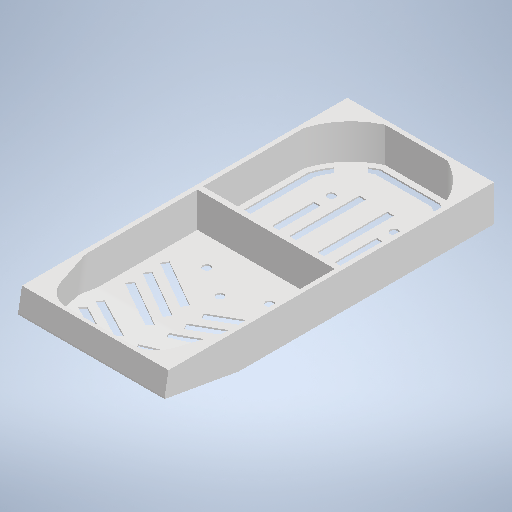
# Autodesk Inventor part: sole_paint_support
Saved by Autodesk Inventor 2026.1 (Build 301233020, 233B)
## iProperties
Created: 2026-02-24
Part Number: sole_paint_support
Material: 一般
Document SubType Name: Modeling
Designer: hibik
Density: 1 g/cm^3
Appearance: 既定
Author: hibik
Autodesk Inventor part; units mm, degrees
ref_plane "YZ Plane" through (0, 0, 0) normal (1, 0, 0) x (0, 1, 0)
ref_plane "XZ Plane" through (0, 0, 0) normal (0, 1, 0) x (-1, 0, 0)
ref_plane "XY Plane" through (0, 0, 0) normal (0, 0, 1) x (1, 0, 0)
sketch "スケッチ1" plane through (0, 0, 0) normal (0, 1, 0) x (-1, 0, 0)
  line L0 (-15.856406, 24.133975) -> (-5.024845, 30.387579)
  line L1 (5.024845, 30.387579) -> (-5.024845, 30.387579)
  line L2 (5.024845, 30.387579) -> (15.856406, 24.133975)
  line L3 (15.856406, 24.133975) -> (16.856406, 25.866025)
  line L4 (16.856406, 25.866025) -> (9.024845, 30.387579)
  line L5 (19, 30.387579) -> (9.024845, 30.387579)
  line L6 (19, 30.387579) -> (19, 3)
  line L7 (19, 3) -> (-19, 3)
  line L8 (-19, 3) -> (-19, 30.387579)
  line L9 (-9.024845, 30.387579) -> (-19, 30.387579)
  line L10 (-9.024845, 30.387579) -> (-16.856406, 25.866025)
  line L11 (-16.856406, 25.866025) -> (-15.856406, 24.133975)
  line L12 (2, 22.133975) -> (15.856406, 14.133975)
  line L13 (15.856406, 14.133975) -> (16.856406, 15.866025)
  line L14 (16.856406, 15.866025) -> (3, 23.866025)
  line L15 (3, 23.866025) -> (2, 22.133975)
  line L16 (2, 27.133975) -> (15.856406, 19.133975)
  line L17 (15.856406, 19.133975) -> (16.856406, 20.866025)
  line L18 (16.856406, 20.866025) -> (3, 28.866025)
  line L19 (3, 28.866025) -> (2, 27.133975)
  line L20 (-16.856406, 15.866025) -> (-15.856406, 14.133975)
  line L21 (-15.856406, 14.133975) -> (-2, 22.133975)
  line L22 (-2, 22.133975) -> (-3, 23.866025)
  line L23 (-3, 23.866025) -> (-16.856406, 15.866025)
  line L24 (-16.856406, 20.866025) -> (-15.856406, 19.133975)
  line L25 (-15.856406, 19.133975) -> (-2, 27.133975)
  line L26 (-2, 27.133975) -> (-3, 28.866025)
  line L27 (-3, 28.866025) -> (-16.856406, 20.866025)
  circle A0 centre (0, 15.5) radius 2.5
  circle A1 centre (-9, 10.307692) radius 2.5
  circle A2 centre (9, 10.307692) radius 2.5
  line L28 (19, -28.244998) -> (19, 0)
  arc A3 (8.717798, -40) -> (19, -28.244998) centre (0, -22) ccw
  line L29 (8.717798, -40) -> (-8.717798, -40)
  arc A4 (-19, -28.244998) -> (-8.717798, -40) centre (0, -22) ccw
  line L30 (-19, -28.244998) -> (-19, 0)
  line L31 (-19, 0) -> (19, 0)
  circle A5 centre (9, -25.384615) radius 2.5
  circle A6 centre (-9, -25.384615) radius 2.5
  circle A7 centre (-9, -4.615385) radius 2.5
  circle A8 centre (9, -4.615385) radius 2.5
  line L32 (-10, -21.384615) -> (-8, -21.384615)
  line L33 (-8, -21.384615) -> (-8, -8.615385)
  line L34 (-8, -8.615385) -> (-10, -8.615385)
  line L35 (-10, -8.615385) -> (-10, -21.384615)
  line L36 (18.05, -27.932748) -> (18.05, -1)
  line L37 (18.05, -1) -> (16.05, -1)
  line L38 (16.05, -1) -> (16.05, -27.603347)
  arc A9 (14.238164, -31.288417) -> (16.05, -27.603347) centre (0, -22) ccw
  line L39 (8, -37) -> (-8, -37)
  arc A10 (-16.05, -27.603347) -> (-14.238164, -31.288417) centre (0, -22) ccw
  line L40 (-16.05, -27.603347) -> (-16.05, -1)
  line L41 (-16.05, -1) -> (-18.05, -1)
  line L42 (-18.05, -1) -> (-18.05, -27.932748)
  arc A11 (15.679986, -32.730239) -> (18.05, -27.932748) centre (0, -22) ccw
  line L43 (-8.485281, -39) -> (8.485281, -39)
  arc A12 (-18.05, -27.932748) -> (-15.679986, -32.730239) centre (0, -22) ccw
  line L44 (-3, -1) -> (-5, -1)
  line L45 (-5, -1) -> (-5, -29.421937)
  line L46 (-5, -29.421937) -> (-3, -29.421937)
  line L47 (-3, -29.421937) -> (-3, -1)
  line L48 (8, -21.384615) -> (10, -21.384615)
  line L49 (10, -21.384615) -> (10, -8.615385)
  line L50 (10, -8.615385) -> (8, -8.615385)
  line L51 (8, -8.615385) -> (8, -21.384615)
  line L52 (5, -1) -> (3, -1)
  line L53 (3, -1) -> (3, -29.421937)
  line L54 (3, -29.421937) -> (5, -29.421937)
  line L55 (5, -29.421937) -> (5, -1)
  line L56 (21, 52.387579) -> (-21, 52.387579)
  line L57 (-21, 52.387579) -> (-21, -42)
  line L58 (-21, -42) -> (21, -42)
  line L59 (21, -42) -> (21, 52.387579)
  line L60 (9.024845, 30.387579) -> (-9.024845, 30.387579)
  line L61 (15.679986, -32.730239) -> (14.238164, -31.288417)
  line L62 (-15.679986, -32.730239) -> (-14.238164, -31.288417)
  line L63 (9.288417, -36.238164) -> (10.730239, -37.679986)
  arc A13 (8, -37) -> (9.288417, -36.238164) centre (0, -22) ccw
  arc A14 (-9.288417, -36.238164) -> (-8, -37) centre (0, -22) ccw
  line L64 (-9.288417, -36.238164) -> (-10.730239, -37.679986)
  arc A15 (-10.730239, -37.679986) -> (-8.485281, -39) centre (0, -22) ccw
  arc A16 (8.485281, -39) -> (10.730239, -37.679986) centre (0, -22) ccw
  point P0 (0, 0)
  point P1 (0, 52.387579)
  dimension "d0" = 2
  dimension "d1" = 2
  dimension "d2" = 22
  constraints: 10 end point, 2 horizontal, 2 parallel, 1 midpoint, 1 perpendicular, 1 vertical alignment
  measures "d0" distance between parallel lines of L58 L29
  measures "d1" distance between parallel lines of L57 L8
  measures "d2" distance between parallel lines of L56 L9
extrude "押し出し1" add sketch "スケッチ1" against normal blind 0.4 contours L0 L1 L2 L3 L4 L5 L6 L7 L8 L9 L10 L11 | A0 | A1 | A2 | A3 L29 A4 L30 L31 L28 | A5 | A6 | A7 | A8 | L59 L58 L57 L56
sketch "スケッチ2" plane through (0, 0, 0) normal (1, 0, 0) x (0, 1, 0)
  line L0 (2.641813, 45.982466) -> (1.055373, 36.985318)
  line L1 (0.670986, 34.805353) -> (1.055373, 36.985318)
  line L2 (0.670986, 34.805353) -> (0.106346, 31.603117)
  arc A0 (0.106346, 31.603117) -> (0, 30.387579) centre (7, 30.387579) ccw
  line L3 (2.641813, 45.982466) -> (3.472964, 50.696155)
  line L4 (0, 52.387579) -> (0, -42)
  line L5 (0, 52.387579) -> (3.771207, 52.387579)
  line L6 (3.771207, 52.387579) -> (3.472964, 50.696155)
  point P0 (0, 0)
  constraints: 4 end point, 1 collinear, 1 horizontal
extrude "押し出し2" add sketch "スケッチ2" along normal mid plane 42
sketch "スケッチ3" plane through (21, -0.4, 52.387579) normal (1, 0, 0) x (0, 0, -1)
  line L0 (20.784463, 0.506346) -> (0, 4.171207)
  line L1 (21.352584, 0) -> (0, 3.765037)
  line L2 (94.387579, 0) -> (0, 0)
  line L3 (0, 4.171207) -> (0, 0)
  point P0 (52.387579, 0.4)
  dimension "d7" = 0.4
  constraints: 2 end point, 2 point on line, 1 parallel
  measures "d7" distance between parallel lines of L1 L0
extrude "押し出し3" cut sketch "スケッチ3" against normal through all
sketch "スケッチ4" plane through (-21, -0.4, 31.034995) normal (0, -0.9848078, 0.1736482) x (1, 0, 0)
  line L0 (18, 16.88502) -> (19, 15.15297)
  line L1 (19, 15.15297) -> (6, 7.647416)
  line L2 (6, 7.647416) -> (5, 9.379467)
  line L3 (5, 9.379467) -> (18, 16.88502)
  line L4 (36, 7.647416) -> (23, 15.15297)
  line L5 (23, 15.15297) -> (24, 16.88502)
  line L6 (24, 16.88502) -> (37, 9.379467)
  line L7 (37, 9.379467) -> (36, 7.647416)
  line L8 (37, 4.379467) -> (36, 2.647416)
  line L9 (36, 2.647416) -> (23, 10.15297)
  line L10 (23, 10.15297) -> (24, 11.88502)
  line L11 (24, 11.88502) -> (37, 4.379467)
  line L12 (19, 10.15297) -> (6, 2.647416)
  line L13 (6, 2.647416) -> (5, 4.379467)
  line L14 (5, 4.379467) -> (18, 11.88502)
  line L15 (18, 11.88502) -> (19, 10.15297)
  line L16 (23.919473, 0.647416) -> (23, 1.186463)
  line L17 (23, 1.186463) -> (24, 2.945234)
  line L18 (24, 2.945234) -> (27.919473, 0.647416)
  line L19 (40, 0.647416) -> (27.919473, 0.647416)
  line L20 (40, 3.899052) -> (40, 0.647416)
  arc A0 (40, 3.899052) -> (39.640783, 6.112646) centre (33, 3.899052) ccw
  line L21 (36.595469, 15.24859) -> (39.640783, 6.112646)
  arc A1 (36.595469, 15.24859) -> (29.954685, 20.034995) centre (29.954685, 13.034995) ccw
  line L22 (29.954685, 20.034995) -> (12.045315, 20.034995)
  arc A2 (12.045315, 20.034995) -> (5.404531, 15.24859) centre (12.045315, 13.034995) ccw
  line L23 (2.359217, 6.112646) -> (5.404531, 15.24859)
  arc A3 (2.359217, 6.112646) -> (2, 3.899052) centre (9, 3.899052) ccw
  line L24 (2, 0.647416) -> (2, 3.899052)
  line L25 (14.080527, 0.647416) -> (2, 0.647416)
  line L26 (14.080527, 0.647416) -> (18, 2.945234)
  line L27 (18, 2.945234) -> (19, 1.186463)
  line L28 (19, 1.186463) -> (18.080527, 0.647416)
  line L29 (23.919473, 0.647416) -> (18.080527, 0.647416)
  line L30 (11.975155, -0.63758) -> (15.975155, -0.63758)
  line L31 (26.024845, -0.63758) -> (30.024845, -0.63758)
  line L32 (26.024845, -0.63758) -> (23.919473, 0.647416)
  line L33 (30.024845, -0.63758) -> (27.919473, 0.647416)
  line L34 (18.080527, 0.647416) -> (15.975155, -0.63758)
  line L35 (4.143594, -5.090442) -> (11.975155, -0.63758)
  line L36 (11.975155, -0.63758) -> (14.080527, 0.647416)
  point P0 (21, -30.494045)
  constraints: 8 end point
extrude "押し出し4" cut sketch "スケッチ4" against normal through all contours L0 L1 L2 L3 | L4 L5 L6 L7 | L8 L9 L10 L11 | L12 L13 L14 L15 | L16 L17 L18 L33 L31 L32 | L34 L30 L36 L26 L27 L28
sketch "スケッチ5" plane through (0, 0, 0) normal (0, 1, 0) x (1, 0, 0)
  line L0 (-19, 28.244998) -> (-19, 0)
  line L1 (-19, 0) -> (19, 0)
  line L2 (19, 0) -> (19, 28.244998)
  arc A0 (19, 28.244998) -> (8.717798, 40) centre (0, 22) ccw
  line L3 (8.717798, 40) -> (-8.717798, 40)
  arc A1 (-8.717798, 40) -> (-19, 28.244998) centre (0, 22) ccw
  circle A2 centre (9, 25.384615) radius 0.8
  circle A3 centre (-9, 25.384615) radius 0.8
  circle A4 centre (9, 4.615385) radius 0.8
  circle A5 centre (-9, 4.615385) radius 0.8
  line L4 (19, -30.037625) -> (-19, -30.037625)
  line L5 (19, -30.037625) -> (19, -3)
  line L6 (19, -3) -> (-19, -3)
  line L7 (-19, -3) -> (-19, -30.037625)
  circle A6 centre (-9, -10.307692) radius 0.8
  circle A7 centre (9, -10.307692) radius 0.8
  circle A8 centre (0, -15.5) radius 0.8
  arc A9 (19.7, 28.356099) -> (8.876936, 40.7) centre (0, 22) ccw
  line L8 (19.7, 28.356099) -> (19.7, -0.7)
  line L9 (19.7, -0.7) -> (-19.7, -0.7)
  line L10 (-19.7, -0.7) -> (-19.7, 28.356099)
  arc A10 (-8.876936, 40.7) -> (-19.7, 28.356099) centre (0, 22) ccw
  line L11 (-8.876936, 40.7) -> (8.876936, 40.7)
  line L12 (19.7, -2.3) -> (19.7, -30.737625)
  line L13 (19.7, -30.737625) -> (-19.7, -30.737625)
  line L14 (-19.7, -30.737625) -> (-19.7, -2.3)
  line L15 (-19.7, -2.3) -> (19.7, -2.3)
  line L16 (-5, 1) -> (-5, 29.421937)
  line L17 (-5, 29.421937) -> (-3, 29.421937)
  line L18 (-3, 29.421937) -> (-3, 1)
  line L19 (-3, 1) -> (-5, 1)
  line L20 (-8, 21.384615) -> (-8, 8.615385)
  line L21 (-8, 8.615385) -> (-10, 8.615385)
  line L22 (-10, 8.615385) -> (-10, 21.384615)
  line L23 (-10, 21.384615) -> (-8, 21.384615)
  line L24 (3, 1) -> (3, 29.421937)
  line L25 (3, 29.421937) -> (5, 29.421937)
  line L26 (5, 29.421937) -> (5, 1)
  line L27 (5, 1) -> (3, 1)
  line L28 (10, 21.384615) -> (10, 8.615385)
  line L29 (10, 8.615385) -> (8, 8.615385)
  line L30 (8, 8.615385) -> (8, 21.384615)
  line L31 (8, 21.384615) -> (10, 21.384615)
  line L32 (16.856406, -20.866025) -> (3, -28.866025)
  line L33 (3, -28.866025) -> (2, -27.133975)
  line L34 (2, -27.133975) -> (15.856406, -19.133975)
  line L35 (15.856406, -19.133975) -> (16.856406, -20.866025)
  line L36 (16.856406, -15.866025) -> (3, -23.866025)
  line L37 (3, -23.866025) -> (2, -22.133975)
  line L38 (2, -22.133975) -> (15.856406, -14.133975)
  line L39 (15.856406, -14.133975) -> (16.856406, -15.866025)
  line L40 (-2, -27.133975) -> (-3, -28.866025)
  line L41 (-3, -28.866025) -> (-16.856406, -20.866025)
  line L42 (-16.856406, -20.866025) -> (-15.856406, -19.133975)
  line L43 (-15.856406, -19.133975) -> (-2, -27.133975)
  line L44 (-2, -22.133975) -> (-3, -23.866025)
  line L45 (-3, -23.866025) -> (-16.856406, -15.866025)
  line L46 (-16.856406, -15.866025) -> (-15.856406, -14.133975)
  line L47 (-15.856406, -14.133975) -> (-2, -22.133975)
  line L48 (-5.147008, -30.317049) -> (-5.024845, -30.317049)
  line L49 (-5.024845, -30.317049) -> (-4.911041, -30.387579)
  line L50 (4.911041, -30.387579) -> (-4.911041, -30.387579)
  line L51 (4.911041, -30.387579) -> (5.024845, -30.317049)
  line L52 (5.024845, -30.317049) -> (5.147008, -30.317049)
  line L53 (5.147008, -30.317049) -> (15.856406, -24.133975)
  line L54 (15.856406, -24.133975) -> (16.856406, -25.866025)
  line L55 (16.856406, -25.866025) -> (9.024845, -30.387579)
  line L56 (21, -30.387579) -> (9.024845, -30.387579)
  line L57 (21, -30.387579) -> (21, 42)
  line L58 (21, 42) -> (-21, 42)
  line L59 (-21, 42) -> (-21, -30.387579)
  line L60 (-9.024845, -30.387579) -> (-21, -30.387579)
  line L61 (-9.024845, -30.387579) -> (-16.856406, -25.866025)
  line L62 (-16.856406, -25.866025) -> (-15.856406, -24.133975)
  line L63 (-15.856406, -24.133975) -> (-5.147008, -30.317049)
  point P0 (0, 0)
  point P1 (19.7, -30.387579)
  point P2 (-19.7, -30.387579)
  dimension "d12" = 0.7
  dimension "d13" = 0.7
  constraints: 16 end point, 4 point on circle, 2 centre point, 8 other
  measures "d12" radial gap between concentric circles of A0 A9
  measures "d13" distance between parallel lines of L5 L12
extrude "押し出し5" add sketch "スケッチ5" along normal blind 10 contours L12 L15 L14 L60 L59 L58 L57 L56
sketch "スケッチ6" plane through (-21, 3.771207, 52.387579) normal (0, 0.9848078, -0.1736482) x (1, 0, 0)
  line L0 (2, 20.755142) -> (40, 20.755142)
  line L1 (2, 17.853461) -> (2, 20.755142)
  arc A0 (2, 17.853461) -> (2.359217, 15.639867) centre (9, 17.853461) ccw
  line L2 (5.404531, 6.503923) -> (2.359217, 15.639867)
  arc A1 (5.404531, 6.503923) -> (12.045315, 1.717517) centre (12.045315, 8.717517) ccw
  line L3 (29.954685, 1.717517) -> (12.045315, 1.717517)
  arc A2 (29.954685, 1.717517) -> (36.595469, 6.503923) centre (29.954685, 8.717517) ccw
  line L4 (39.640783, 15.639867) -> (36.595469, 6.503923)
  arc A3 (39.640783, 15.639867) -> (40, 17.853461) centre (33, 17.853461) ccw
  line L5 (40, 20.755142) -> (40, 17.853461)
  arc A4 (29.954685, 1.017517) -> (37.259547, 6.282563) centre (29.954685, 8.717517) ccw
  line L6 (29.954685, 1.017517) -> (12.045315, 1.017517)
  arc A5 (4.740453, 6.282563) -> (12.045315, 1.017517) centre (12.045315, 8.717517) ccw
  line L7 (4.740453, 6.282563) -> (1.695139, 15.418507)
  arc A6 (1.3, 17.853461) -> (1.695139, 15.418507) centre (9, 17.853461) ccw
  line L8 (1.3, 17.853461) -> (1.3, 21.455142)
  line L9 (1.3, 21.455142) -> (40.7, 21.455142)
  line L10 (40.7, 21.455142) -> (40.7, 17.853461)
  arc A7 (40.304861, 15.418507) -> (40.7, 17.853461) centre (33, 17.853461) ccw
  line L11 (40.304861, 15.418507) -> (37.259547, 6.282563)
  line L12 (18, 18.807279) -> (14.080527, 21.105097)
  line L13 (14.080527, 21.105097) -> (0, 21.105097)
  line L14 (0, 0) -> (0, 21.105097)
  line L15 (0, 0) -> (42, 0)
  line L16 (42, 21.105097) -> (42, 0)
  line L17 (42, 21.105097) -> (27.919473, 21.105097)
  line L18 (27.919473, 21.105097) -> (24, 18.807279)
  line L19 (24, 18.807279) -> (23, 20.566049)
  line L20 (23, 20.566049) -> (23.919473, 21.105097)
  line L21 (23.919473, 21.105097) -> (18.080527, 21.105097)
  line L22 (18.080527, 21.105097) -> (19, 20.566049)
  line L23 (19, 20.566049) -> (18, 18.807279)
  line L24 (5, 17.373046) -> (6, 19.105097)
  line L25 (6, 19.105097) -> (19, 11.599543)
  line L26 (19, 11.599543) -> (18, 9.867492)
  line L27 (18, 9.867492) -> (5, 17.373046)
  line L28 (24, 4.867492) -> (23, 6.599543)
  line L29 (23, 6.599543) -> (36, 14.105097)
  line L30 (36, 14.105097) -> (37, 12.373046)
  line L31 (37, 12.373046) -> (24, 4.867492)
  line L32 (6, 14.105097) -> (19, 6.599543)
  line L33 (19, 6.599543) -> (18, 4.867492)
  line L34 (18, 4.867492) -> (5, 12.373046)
  line L35 (5, 12.373046) -> (6, 14.105097)
  line L36 (23, 11.599543) -> (36, 19.105097)
  line L37 (36, 19.105097) -> (37, 17.373046)
  line L38 (37, 17.373046) -> (24, 9.867492)
  line L39 (24, 9.867492) -> (23, 11.599543)
  point P0 (21, 52.246558)
  point P1 (1.3, 21.105097)
  point P2 (40.7, 21.105097)
  dimension "d16" = 0.7
  constraints: 12 end point, 8 point on circle, 4 centre point, 9 other
  measures "d16" distance between parallel lines of L4 L11
extrude "押し出し6" add sketch "スケッチ6" along normal blind 10 contours L8 A6 L7 A5 L6 A4 L11 A7 L10 L17 L16 L15 L14 L13
sketch "スケッチ7" plane through (-21, -0.4, -42) normal (-1, 0, 0) x (0, 0, 1)
  line L0 (73.603117, 0.506346) -> (72.387579, 7.4)
  arc A0 (72.387579, 0.4) -> (73.603117, 0.506346) centre (72.387579, 7.4) ccw
  line L1 (72.387579, 0.4) -> (72.387579, 7.4)
  line L2 (73.603117, 0.506346) -> (72.387579, 7.4)
  line L3 (94.387579, 4.171207) -> (92.651098, 14.019285)
  line L4 (72.125113, 10.4) -> (92.651098, 14.019285)
  line L5 (0, 10.4) -> (72.125113, 10.4)
  line L6 (0, 0) -> (0, 10.4)
  line L7 (73.034995, 0) -> (0, 0)
  line L8 (73.034995, 0) -> (94.387579, 3.765037)
  line L9 (94.387579, 3.765037) -> (94.387579, 4.171207)
  point P0 (42, 0.4)
extrude "押し出し7" add sketch "スケッチ7" against normal up to surface (1.3 mm away) contours A0 L1 L0
sketch "スケッチ8" plane through (21, -0.4, 31.034995) normal (1, 0, 0) x (0, 0, -1)
  line L0 (-21.352584, 4.171207) -> (-21.352584, 3.765037)
  line L1 (-21.352584, 3.765037) -> (0, 0)
  line L2 (73.034995, 0) -> (0, 0)
  line L3 (73.034995, 0) -> (73.034995, 10.4)
  line L4 (0.909882, 10.4) -> (73.034995, 10.4)
  line L5 (-19.616102, 14.019285) -> (0.909882, 10.4)
  line L6 (-21.352584, 4.171207) -> (-19.616102, 14.019285)
  line L7 (-0.568121, 0.506346) -> (0.647416, 7.4)
  line L8 (0.647416, 0.4) -> (0.647416, 7.4)
  arc A0 (-0.568121, 0.506346) -> (0.647416, 0.4) centre (0.647416, 7.4) ccw
  point P0 (31.034995, 0.4)
extrude "押し出し8" add sketch "スケッチ8" against normal up to surface (1.3 mm away) contours L7 L8 A0
sketch "スケッチ9" plane through (0, 10, 0) normal (0, 1, 0) x (1, 0, 0)
  line L0 (50.426024, -14.988478) -> (-44.417108, -14.988478)
  line L1 (-44.417108, -14.988478) -> (-44.417108, -64.562339)
  line L2 (-44.417108, -64.562339) -> (50.426024, -64.562339)
  line L3 (50.426024, -64.562339) -> (50.426024, -14.988478)
  point P0 (0, 0)
  constraints: 8 end point, 2 parallel, 1 horizontal, 1 perpendicular
extrude "押し出し9" cut sketch "スケッチ9" along normal through all
sketch "スケッチ10" plane through (0, -0.4, 0) normal (0, -1, 0) x (1, 0, 0)
  circle A0 centre (9, -4.615385) radius 2.5
  circle A1 centre (-9, -4.615385) radius 2.5
  circle A2 centre (-9, -25.384615) radius 2.5
  circle A3 centre (9, -25.384615) radius 2.5
  circle A4 centre (9, 10.307692) radius 2.5
  circle A5 centre (-9, 10.307692) radius 2.5
  circle A6 centre (0, 15.5) radius 2.5
  circle A7 centre (9, -25.384615) radius 1.15
  circle A8 centre (-9, -25.384615) radius 1.15
  circle A9 centre (9, -4.615385) radius 1.15
  circle A10 centre (-9, -4.615385) radius 1.15
  circle A11 centre (-9, 10.307692) radius 1.15
  circle A12 centre (9, 10.307692) radius 1.15
  circle A13 centre (0, 15.5) radius 1.15
  point P0 (0, 0)
extrude "押し出し10" cut sketch "スケッチ10" against normal through all contours A7 | A8 | A9 | A10 | A11 | A12 | A13
equation "\"d1\" = d0"
